Autodesk Fusion 360 part; units mm, degrees
(part 18 of 21)
  spline S78 degree 5 poles (9.9022, -20.7593) (9.9022, -20.752) (9.9024, -20.7374) (9.9025, -20.7155) (9.9026, -20.6864) (9.9026, -20.65) (9.9024, -20.6137) (9.9021, -20.5774) (9.9017, -20.5411) (9.9011, -20.5049) (9.9004, -20.4687) (9.8996, -20.4326) (9.8986, -20.3965) (9.8975, -20.3604) (9.8963, -20.3244) (9.8949, -20.2885) (9.8934, -20.2525) (9.8917, -20.2167) (9.8899, -20.1808) (9.8879, -20.145) (9.8858, -20.1093) (9.8836, -20.0736) (9.8812, -20.038) (9.8786, -20.0024) (9.8759, -19.9668) (9.8731, -19.9313) (9.8701, -19.8959) (9.867, -19.8605) (9.8637, -19.8252) (9.8602, -19.7899) (9.8566, -19.7547) (9.8529, -19.7195) (9.8489, -19.6844) (9.8449, -19.6493) (9.8406, -19.6143) (9.8362, -19.5794) (9.8316, -19.5445) (9.8269, -19.5097) (9.822, -19.4749) (9.8169, -19.4402) (9.8117, -19.4056) (9.8063, -19.3711) (9.8007, -19.3366) (9.7949, -19.3021) (9.789, -19.2678) (9.7828, -19.2335) (9.7765, -19.1993) (9.77, -19.1652) (9.7633, -19.1311) (9.7564, -19.0972) (9.7493, -19.0633) (9.742, -19.0295) (9.7345, -18.9957) (9.7268, -18.9621) (9.7189, -18.9286) (9.7108, -18.8951) (9.7024, -18.8618) (9.6938, -18.8285) (9.685, -18.7954) (9.6759, -18.7624) (9.6665, -18.7294) (9.6569, -18.6966) (9.6471, -18.6639) (9.637, -18.6313) (9.6266, -18.5989) (9.6158, -18.5666) (9.6066, -18.54) (9.5994, -18.5199) (9.5944, -18.5063) (9.5917, -18.499) (9.5913, -18.4981) knots -1 -1 -1 -1 -1 -1 -0.98571429 -0.97142857 -0.95714286 -0.94285714 -0.92857143 -0.91428571 -0.9 -0.88571429 -0.87142857 -0.85714286 -0.84285714 -0.82857143 -0.81428571 -0.8 -0.78571429 -0.77142857 -0.75714286 -0.74285714 -0.72857143 -0.71428571 -0.7 -0.68571429 -0.67142857 -0.65714286 -0.64285714 -0.62857143 -0.61428571 -0.6 -0.58571429 -0.57142857 -0.55714286 -0.54285714 -0.52857143 -0.51428571 -0.5 -0.48571429 -0.47142857 -0.45714286 -0.44285714 -0.42857143 -0.41428571 -0.4 -0.38571429 -0.37142857 -0.35714286 -0.34285714 -0.32857143 -0.31428571 -0.3 -0.28571429 -0.27142857 -0.25714286 -0.24285714 -0.22857143 -0.21428571 -0.2 -0.18571429 -0.17142857 -0.15714286 -0.14285714 -0.12857143 -0.11428571 -0.1 -0.08571429 -0.07142857 -0.06937658 -0.06937658 -0.06937658 -0.06937658 -0.06937658 -0.06937658
  spline S79 degree 3 poles (9.6386, -18.3746) (9.6271, -18.3807) (9.6168, -18.3889) (9.6001, -18.4089) (9.5937, -18.4204) (9.5864, -18.4434) (9.5848, -18.4545) (9.5853, -18.4767) (9.5875, -18.4877) (9.5913, -18.4981) knots 0 0 0 0 0.003906 0.003906 0.007813 0.007813 0.011148 0.011148 0.014483 0.014483 0.014483 0.014483
  arc A70 (9.6386, -18.3746) -> (10.2467, -18.0426) centre (0, 0) ccw
  spline S80 degree 3 poles (10.3761, -18.0696) (10.3683, -18.0592) (10.3585, -18.0504) (10.3362, -18.037) (10.3238, -18.0326) (10.2999, -18.029) (10.2887, -18.0292) (10.2669, -18.0332) (10.2564, -18.0371) (10.2467, -18.0426) knots 0 0 0 0 0.003906 0.003906 0.007813 0.007813 0.011148 0.011148 0.014483 0.014483 0.014483 0.014483
  spline S81 degree 5 poles (10.3761, -18.0696) (10.3767, -18.0704) (10.3813, -18.0766) (10.3901, -18.0882) (10.4031, -18.1051) (10.4205, -18.1272) (10.4419, -18.1537) (10.4635, -18.18) (10.4855, -18.2061) (10.5077, -18.2321) (10.5301, -18.2579) (10.5527, -18.2835) (10.5756, -18.3091) (10.5987, -18.3344) (10.622, -18.3596) (10.6455, -18.3847) (10.6693, -18.4096) (10.6932, -18.4344) (10.7173, -18.4591) (10.7417, -18.4836) (10.7662, -18.508) (10.7908, -18.5323) (10.8157, -18.5565) (10.8407, -18.5805) (10.8659, -18.6045) (10.8913, -18.6283) (10.9168, -18.652) (10.9425, -18.6755) (10.9683, -18.699) (10.9943, -18.7223) (11.0204, -18.7456) (11.0467, -18.7687) (11.0732, -18.7917) (11.0998, -18.8147) (11.1265, -18.8375) (11.1534, -18.8602) (11.1804, -18.8828) (11.2075, -18.9052) (11.2348, -18.9276) (11.2622, -18.9499) (11.2898, -18.9721) (11.3175, -18.9942) (11.3453, -19.0161) (11.3732, -19.038) (11.4013, -19.0598) (11.4295, -19.0815) (11.4578, -19.1031) (11.4863, -19.1245) (11.5149, -19.1459) (11.5435, -19.1672) (11.5724, -19.1884) (11.6013, -19.2095) (11.6303, -19.2305) (11.6595, -19.2514) (11.6888, -19.2722) (11.7182, -19.2929) (11.7477, -19.3135) (11.7773, -19.334) (11.807, -19.3544) (11.8369, -19.3748) (11.8668, -19.395) (11.8969, -19.4152) (11.927, -19.4352) (11.9573, -19.4552) (11.9877, -19.475) (12.0182, -19.4948) (12.0488, -19.5145) (12.0733, -19.5302) (12.0918, -19.5419) (12.1041, -19.5497) (12.1103, -19.5535) knots 0.06937658 0.06937658 0.06937658 0.06937658 0.06937658 0.06937658 0.07142857 0.08571429 0.1 0.11428571 0.12857143 0.14285714 0.15714286 0.17142857 0.18571429 0.2 0.21428571 0.22857143 0.24285714 0.25714286 0.27142857 0.28571429 0.3 0.31428571 0.32857143 0.34285714 0.35714286 0.37142857 0.38571429 0.4 0.41428571 0.42857143 0.44285714 0.45714286 0.47142857 0.48571429 0.5 0.51428571 0.52857143 0.54285714 0.55714286 0.57142857 0.58571429 0.6 0.61428571 0.62857143 0.64285714 0.65714286 0.67142857 0.68571429 0.7 0.71428571 0.72857143 0.74285714 0.75714286 0.77142857 0.78571429 0.8 0.81428571 0.82857143 0.84285714 0.85714286 0.87142857 0.88571429 0.9 0.91428571 0.92857143 0.94285714 0.95714286 0.97142857 0.98571429 1 1 1 1 1 1
  arc A71 (12.1103, -19.5535) -> (12.7557, -19.1387) centre (0, 0) ccw
  spline S82 degree 5 poles (12.7557, -19.1387) (12.7548, -19.1315) (12.7528, -19.1171) (12.7498, -19.0954) (12.7458, -19.0665) (12.7406, -19.0305) (12.7352, -18.9946) (12.7298, -18.9587) (12.7242, -18.9229) (12.7185, -18.8871) (12.7127, -18.8514) (12.7067, -18.8158) (12.7006, -18.7802) (12.6944, -18.7446) (12.688, -18.7092) (12.6815, -18.6738) (12.6749, -18.6384) (12.6681, -18.6032) (12.6612, -18.5679) (12.6542, -18.5328) (12.647, -18.4977) (12.6397, -18.4627) (12.6323, -18.4278) (12.6247, -18.3929) (12.617, -18.3581) (12.6091, -18.3234) (12.6011, -18.2887) (12.593, -18.2541) (12.5847, -18.2196) (12.5763, -18.1852) (12.5677, -18.1509) (12.5589, -18.1166) (12.5501, -18.0824) (12.541, -18.0483) (12.5319, -18.0142) (12.5225, -17.9803) (12.513, -17.9464) (12.5034, -17.9126) (12.4936, -17.8789) (12.4836, -17.8453) (12.4735, -17.8117) (12.4633, -17.7783) (12.4528, -17.745) (12.4422, -17.7117) (12.4314, -17.6786) (12.4205, -17.6455) (12.4094, -17.6125) (12.3981, -17.5797) (12.3866, -17.5469) (12.3749, -17.5143) (12.3631, -17.4818) (12.351, -17.4493) (12.3388, -17.417) (12.3264, -17.3848) (12.3138, -17.3527) (12.301, -17.3208) (12.288, -17.289) (12.2747, -17.2573) (12.2612, -17.2258) (12.2475, -17.1944) (12.2336, -17.1631) (12.2194, -17.132) (12.205, -17.101) (12.1904, -17.0702) (12.1755, -17.0396) (12.1602, -17.0092) (12.1473, -16.9841) (12.1374, -16.9653) (12.1304, -16.9525) (12.1267, -16.9457) (12.1263, -16.9448) knots -1 -1 -1 -1 -1 -1 -0.98571429 -0.97142857 -0.95714286 -0.94285714 -0.92857143 -0.91428571 -0.9 -0.88571429 -0.87142857 -0.85714286 -0.84285714 -0.82857143 -0.81428571 -0.8 -0.78571429 -0.77142857 -0.75714286 -0.74285714 -0.72857143 -0.71428571 -0.7 -0.68571429 -0.67142857 -0.65714286 -0.64285714 -0.62857143 -0.61428571 -0.6 -0.58571429 -0.57142857 -0.55714286 -0.54285714 -0.52857143 -0.51428571 -0.5 -0.48571429 -0.47142857 -0.45714286 -0.44285714 -0.42857143 -0.41428571 -0.4 -0.38571429 -0.37142857 -0.35714286 -0.34285714 -0.32857143 -0.31428571 -0.3 -0.28571429 -0.27142857 -0.25714286 -0.24285714 -0.22857143 -0.21428571 -0.2 -0.18571429 -0.17142857 -0.15714286 -0.14285714 -0.12857143 -0.11428571 -0.1 -0.08571429 -0.07142857 -0.06937658 -0.06937658 -0.06937658 -0.06937658 -0.06937658 -0.06937658
  spline S83 degree 3 poles (12.1555, -16.8159) (12.1449, -16.8235) (12.136, -16.8331) (12.1222, -16.8552) (12.1176, -16.8675) (12.1136, -16.8914) (12.1136, -16.9025) (12.1173, -16.9245) (12.1209, -16.9351) (12.1263, -16.9448) knots 0 0 0 0 0.003906 0.003906 0.007813 0.007813 0.011148 0.011148 0.014483 0.014483 0.014483 0.014483
  arc A72 (12.1555, -16.8159) -> (12.7101, -16.4007) centre (0, 0) ccw
  spline S84 degree 3 poles (12.8421, -16.409) (12.8329, -16.3998) (12.8219, -16.3925) (12.7979, -16.3824) (12.785, -16.3798) (12.7609, -16.3796) (12.7498, -16.3814) (12.7288, -16.3886) (12.7189, -16.3939) (12.7101, -16.4007) knots 0 0 0 0 0.003906 0.003906 0.007813 0.007813 0.011148 0.011148 0.014483 0.014483 0.014483 0.014483
  spline S85 degree 5 poles (12.8421, -16.409) (12.8428, -16.4097) (12.8482, -16.4151) (12.8586, -16.4254) (12.8739, -16.4403) (12.8942, -16.4597) (12.9191, -16.4829) (12.9443, -16.5058) (12.9698, -16.5286) (12.9954, -16.5511) (13.0213, -16.5735) (13.0473, -16.5956) (13.0736, -16.6176) (13.1001, -16.6394) (13.1267, -16.6611) (13.1536, -16.6826) (13.1806, -16.7039) (13.2079, -16.725) (13.2353, -16.746) (13.2628, -16.7668) (13.2905, -16.7875) (13.3184, -16.808) (13.3465, -16.8284) (13.3747, -16.8486) (13.403, -16.8687) (13.4315, -16.8887) (13.4601, -16.9085) (13.4889, -16.9282) (13.5178, -16.9477) (13.5469, -16.9671) (13.576, -16.9864) (13.6054, -17.0056) (13.6348, -17.0246) (13.6644, -17.0435) (13.6941, -17.0623) (13.7239, -17.0809) (13.7539, -17.0994) (13.784, -17.1178) (13.8141, -17.1361) (13.8445, -17.1542) (13.8749, -17.1723) (13.9054, -17.1902) (13.9361, -17.208) (13.9669, -17.2257) (13.9978, -17.2432) (14.0288, -17.2607) (14.0599, -17.278) (14.0911, -17.2952) (14.1224, -17.3123) (14.1538, -17.3293) (14.1854, -17.3462) (14.217, -17.3629) (14.2487, -17.3796) (14.2806, -17.3961) (14.3125, -17.4125) (14.3446, -17.4288) (14.3767, -17.445) (14.4089, -17.4611) (14.4413, -17.4771) (14.4737, -17.493) (14.5062, -17.5088) (14.5388, -17.5244) (14.5715, -17.54) (14.6044, -17.5554) (14.6373, -17.5708) (14.6702, -17.586) (14.7033, -17.6011) (14.7299, -17.6132) (14.7498, -17.6221) (14.7631, -17.6281) (14.7698, -17.631) knots 0.06937658 0.06937658 0.06937658 0.06937658 0.06937658 0.06937658 0.07142857 0.08571429 0.1 0.11428571 0.12857143 0.14285714 0.15714286 0.17142857 0.18571429 0.2 0.21428571 0.22857143 0.24285714 0.25714286 0.27142857 0.28571429 0.3 0.31428571 0.32857143 0.34285714 0.35714286 0.37142857 0.38571429 0.4 0.41428571 0.42857143 0.44285714 0.45714286 0.47142857 0.48571429 0.5 0.51428571 0.52857143 0.54285714 0.55714286 0.57142857 0.58571429 0.6 0.61428571 0.62857143 0.64285714 0.65714286 0.67142857 0.68571429 0.7 0.71428571 0.72857143 0.74285714 0.75714286 0.77142857 0.78571429 0.8 0.81428571 0.82857143 0.84285714 0.85714286 0.87142857 0.88571429 0.9 0.91428571 0.92857143 0.94285714 0.95714286 0.97142857 0.98571429 1 1 1 1 1 1
  arc A73 (14.7698, -17.631) -> (15.3496, -17.1286) centre (0, 0) ccw
  spline S86 degree 5 poles (15.3496, -17.1286) (15.3476, -17.1216) (15.3436, -17.1076) (15.3376, -17.0865) (15.3295, -17.0586) (15.3192, -17.0237) (15.3088, -16.9888) (15.2983, -16.9541) (15.2877, -16.9194) (15.277, -16.8848) (15.2661, -16.8503) (15.2551, -16.8159) (15.244, -16.7815) (15.2328, -16.7472) (15.2215, -16.713) (15.21, -16.6789) (15.1984, -16.6449) (15.1867, -16.6109) (15.1749, -16.5771) (15.1629, -16.5433) (15.1508, -16.5096) (15.1386, -16.476) (15.1263, -16.4425) (15.1138, -16.409) (15.1012, -16.3757) (15.0885, -16.3424) (15.0756, -16.3093) (15.0626, -16.2762) (15.0495, -16.2432) (15.0363, -16.2103) (15.0229, -16.1775) (15.0094, -16.1448) (14.9957, -16.1123) (14.9819, -16.0798) (14.968, -16.0474) (14.9539, -16.0151) (14.9397, -15.9829) (14.9254, -15.9508) (14.9109, -15.9189) (14.8962, -15.887) (14.8814, -15.8553) (14.8665, -15.8236) (14.8514, -15.7921) (14.8362, -15.7607) (14.8208, -15.7294) (14.8053, -15.6983) (14.7896, -15.6672) (14.7737, -15.6363) (14.7577, -15.6055) (14.7415, -15.5749) (14.7252, -15.5444) (14.7086, -15.514) (14.6919, -15.4837) (14.6751, -15.4536) (14.658, -15.4237) (14.6408, -15.3939) (14.6234, -15.3642) (14.6057, -15.3348) (14.5879, -15.3055) (14.5699, -15.2763) (14.5516, -15.2474) (14.5332, -15.2186) (14.5145, -15.19) (14.4957, -15.1616) (14.4765, -15.1334) (14.4571, -15.1054) (14.4408, -15.0825) (14.4282, -15.0653) (14.4196, -15.0536) (14.4149, -15.0474) (14.4143, -15.0466) knots -1 -1 -1 -1 -1 -1 -0.98571429 -0.97142857 -0.95714286 -0.94285714 -0.92857143 -0.91428571 -0.9 -0.88571429 -0.87142857 -0.85714286 -0.84285714 -0.82857143 -0.81428571 -0.8 -0.78571429 -0.77142857 -0.75714286 -0.74285714 -0.72857143 -0.71428571 -0.7 -0.68571429 -0.67142857 -0.65714286 -0.64285714 -0.62857143 -0.61428571 -0.6 -0.58571429 -0.57142857 -0.55714286 -0.54285714 -0.52857143 -0.51428571 -0.5 -0.48571429 -0.47142857 -0.45714286 -0.44285714 -0.42857143 -0.41428571 -0.4 -0.38571429 -0.37142857 -0.35714286 -0.34285714 -0.32857143 -0.31428571 -0.3 -0.28571429 -0.27142857 -0.25714286 -0.24285714 -0.22857143 -0.21428571 -0.2 -0.18571429 -0.17142857 -0.15714286 -0.14285714 -0.12857143 -0.11428571 -0.1 -0.08571429 -0.07142857 -0.06937658 -0.06937658 -0.06937658 -0.06937658 -0.06937658 -0.06937658
  spline S87 degree 3 poles (14.4249, -14.9148) (14.4155, -14.9239) (14.408, -14.9347) (14.3976, -14.9585) (14.3947, -14.9713) (14.3942, -14.9955) (14.3958, -15.0066) (14.4026, -15.0277) (14.4077, -15.0377) (14.4143, -15.0466) knots 0 0 0 0 0.003906 0.003906 0.007813 0.007813 0.011148 0.011148 0.014483 0.014483 0.014483 0.014483
  arc A74 (14.4249, -14.9148) -> (14.9148, -14.4249) centre (0, 0) ccw
  spline S88 degree 3 poles (15.0466, -14.4143) (15.0362, -14.4065) (15.0243, -14.4009) (14.9991, -14.3943) (14.986, -14.3936) (14.9621, -14.3969) (14.9514, -14.4002) (14.9315, -14.4103) (14.9225, -14.4169) (14.9148, -14.4249) knots 0 0 0 0 0.003906 0.003906 0.007813 0.007813 0.011148 0.011148 0.014483 0.014483 0.014483 0.014483
  spline S89 degree 5 poles (15.0466, -14.4143) (15.0474, -14.4149) (15.0536, -14.4196) (15.0653, -14.4282) (15.0825, -14.4408) (15.1054, -14.4571) (15.1334, -14.4765) (15.1616, -14.4957) (15.19, -14.5145) (15.2186, -14.5332) (15.2474, -14.5516) (15.2763, -14.5699) (15.3055, -14.5879) (15.3348, -14.6057) (15.3642, -14.6234) (15.3939, -14.6408) (15.4237, -14.658) (15.4536, -14.6751) (15.4837, -14.6919) (15.514, -14.7086) (15.5444, -14.7252) (15.5749, -14.7415) (15.6055, -14.7577) (15.6363, -14.7737) (15.6672, -14.7896) (15.6983, -14.8053) (15.7294, -14.8208) (15.7607, -14.8362) (15.7921, -14.8514) (15.8236, -14.8665) (15.8553, -14.8814) (15.887, -14.8962) (15.9189, -14.9109) (15.9508, -14.9254) (15.9829, -14.9397) (16.0151, -14.9539) (16.0474, -14.968) (16.0798, -14.9819) (16.1123, -14.9957) (16.1448, -15.0094) (16.1775, -15.0229) (16.2103, -15.0363) (16.2432, -15.0495) (16.2762, -15.0626) (16.3093, -15.0756) (16.3424, -15.0885) (16.3757, -15.1012) (16.409, -15.1138) (16.4425, -15.1263) (16.476, -15.1386) (16.5096, -15.1508) (16.5433, -15.1629) (16.5771, -15.1749) (16.6109, -15.1867) (16.6449, -15.1984) (16.6789, -15.21) (16.713, -15.2215) (16.7472, -15.2328) (16.7815, -15.244) (16.8159, -15.2551) (16.8503, -15.2661) (16.8848, -15.277) (16.9194, -15.2877) (16.9541, -15.2983) (16.9888, -15.3088) (17.0237, -15.3192) (17.0586, -15.3295) (17.0865, -15.3376) (17.1076, -15.3436) (17.1216, -15.3476) (17.1286, -15.3496) knots 0.06937658 0.06937658 0.06937658 0.06937658 0.06937658 0.06937658 0.07142857 0.08571429 0.1 0.11428571 0.12857143 0.14285714 0.15714286 0.17142857 0.18571429 0.2 0.21428571 0.22857143 0.24285714 0.25714286 0.27142857 0.28571429 0.3 0.31428571 0.32857143 0.34285714 0.35714286 0.37142857 0.38571429 0.4 0.41428571 0.42857143 0.44285714 0.45714286 0.47142857 0.48571429 0.5 0.51428571 0.52857143 0.54285714 0.55714286 0.57142857 0.58571429 0.6 0.61428571 0.62857143 0.64285714 0.65714286 0.67142857 0.68571429 0.7 0.71428571 0.72857143 0.74285714 0.75714286 0.77142857 0.78571429 0.8 0.81428571 0.82857143 0.84285714 0.85714286 0.87142857 0.88571429 0.9 0.91428571 0.92857143 0.94285714 0.95714286 0.97142857 0.98571429 1 1 1 1 1 1
  arc A75 (17.1286, -15.3496) -> (17.631, -14.7698) centre (0, 0) ccw
  spline S90 degree 5 poles (17.631, -14.7698) (17.6281, -14.7631) (17.6221, -14.7498) (17.6132, -14.7299) (17.6011, -14.7033) (17.586, -14.6702) (17.5708, -14.6373) (17.5554, -14.6044) (17.54, -14.5715) (17.5244, -14.5388) (17.5088, -14.5062) (17.493, -14.4737) (17.4771, -14.4413) (17.4611, -14.4089) (17.445, -14.3767) (17.4288, -14.3446) (17.4125, -14.3125) (17.3961, -14.2806) (17.3796, -14.2487) (17.3629, -14.217) (17.3462, -14.1854) (17.3293, -14.1538) (17.3123, -14.1224) (17.2952, -14.0911) (17.278, -14.0599) (17.2607, -14.0288) (17.2432, -13.9978) (17.2257, -13.9669) (17.208, -13.9361) (17.1902, -13.9054) (17.1723, -13.8749) (17.1542, -13.8445) (17.1361, -13.8141) (17.1178, -13.784) (17.0994, -13.7539) (17.0809, -13.7239) (17.0623, -13.6941) (17.0435, -13.6644) (17.0246, -13.6348) (17.0056, -13.6054) (16.9864, -13.576) (16.9671, -13.5469) (16.9477, -13.5178) (16.9282, -13.4889) (16.9085, -13.4601) (16.8887, -13.4315) (16.8687, -13.403) (16.8486, -13.3747) (16.8284, -13.3465) (16.808, -13.3184) (16.7875, -13.2905) (16.7668, -13.2628) (16.746, -13.2353) (16.725, -13.2079) (16.7039, -13.1806) (16.6826, -13.1536) (16.6611, -13.1267) (16.6394, -13.1001) (16.6176, -13.0736) (16.5956, -13.0473) (16.5735, -13.0213) (16.5511, -12.9954) (16.5286, -12.9698) (16.5058, -12.9443) (16.4829, -12.9191) (16.4597, -12.8942) (16.4403, -12.8739) (16.4254, -12.8586) (16.4151, -12.8482) (16.4097, -12.8428) (16.409, -12.8421) knots -1 -1 -1 -1 -1 -1 -0.98571429 -0.97142857 -0.95714286 -0.94285714 -0.92857143 -0.91428571 -0.9 -0.88571429 -0.87142857 -0.85714286 -0.84285714 -0.82857143 -0.81428571 -0.8 -0.78571429 -0.77142857 -0.75714286 -0.74285714 -0.72857143 -0.71428571 -0.7 -0.68571429 -0.67142857 -0.65714286 -0.64285714 -0.62857143 -0.61428571 -0.6 -0.58571429 -0.57142857 -0.55714286 -0.54285714 -0.52857143 -0.51428571 -0.5 -0.48571429 -0.47142857 -0.45714286 -0.44285714 -0.42857143 -0.41428571 -0.4 -0.38571429 -0.37142857 -0.35714286 -0.34285714 -0.32857143 -0.31428571 -0.3 -0.28571429 -0.27142857 -0.25714286 -0.24285714 -0.22857143 -0.21428571 -0.2 -0.18571429 -0.17142857 -0.15714286 -0.14285714 -0.12857143 -0.11428571 -0.1 -0.08571429 -0.07142857 -0.06937658 -0.06937658 -0.06937658 -0.06937658 -0.06937658 -0.06937658
  spline S91 degree 3 poles (16.4007, -12.7101) (16.3927, -12.7204) (16.3868, -12.7322) (16.3799, -12.7573) (16.3789, -12.7704) (16.3818, -12.7943) (16.3849, -12.8051) (16.3946, -12.8251) (16.4011, -12.8342) (16.409, -12.8421) knots 0 0 0 0 0.003906 0.003906 0.007813 0.007813 0.011148 0.011148 0.014483 0.014483 0.014483 0.014483
  arc A76 (16.4007, -12.7101) -> (16.8159, -12.1555) centre (0, 0) ccw
  spline S92 degree 3 poles (16.9448, -12.1263) (16.9334, -12.12) (16.9208, -12.1161) (16.895, -12.1132) (16.8819, -12.1143) (16.8587, -12.121) (16.8486, -12.1258) (16.8304, -12.1386) (16.8224, -12.1465) (16.8159, -12.1555) knots 0 0 0 0 0.003906 0.003906 0.007813 0.007813 0.011148 0.011148 0.014483 0.014483 0.014483 0.014483
  spline S93 degree 5 poles (16.9448, -12.1263) (16.9457, -12.1267) (16.9525, -12.1304) (16.9653, -12.1374) (16.9841, -12.1473) (17.0092, -12.1602) (17.0396, -12.1755) (17.0702, -12.1904) (17.101, -12.205) (17.132, -12.2194) (17.1631, -12.2336) (17.1944, -12.2475) (17.2258, -12.2612) (17.2573, -12.2747) (17.289, -12.288) (17.3208, -12.301) (17.3527, -12.3138) (17.3848, -12.3264) (17.417, -12.3388) (17.4493, -12.351) (17.4818, -12.3631) (17.5143, -12.3749) (17.5469, -12.3866) (17.5797, -12.3981) (17.6125, -12.4094) (17.6455, -12.4205) (17.6786, -12.4314) (17.7117, -12.4422) (17.745, -12.4528) (17.7783, -12.4633) (17.8117, -12.4735) (17.8453, -12.4836) (17.8789, -12.4936) (17.9126, -12.5034) (17.9464, -12.513) (17.9803, -12.5225) (18.0142, -12.5319) (18.0483, -12.541) (18.0824, -12.5501) (18.1166, -12.5589) (18.1509, -12.5677) (18.1852, -12.5763) (18.2196, -12.5847) (18.2541, -12.593) (18.2887, -12.6011) (18.3234, -12.6091) (18.3581, -12.617) (18.3929, -12.6247) (18.4278, -12.6323) (18.4627, -12.6397) (18.4977, -12.647) (18.5328, -12.6542) (18.5679, -12.6612) (18.6032, -12.6681) (18.6384, -12.6749) (18.6738, -12.6815) (18.7092, -12.688) (18.7446, -12.6944) (18.7802, -12.7006) (18.8158, -12.7067) (18.8514, -12.7127) (18.8871, -12.7185) (18.9229, -12.7242) (18.9587, -12.7298) (18.9946, -12.7352) (19.0305, -12.7406) (19.0665, -12.7458) (19.0954, -12.7498) (19.1171, -12.7528) (19.1315, -12.7548) (19.1387, -12.7557) knots 0.06937658 0.06937658 0.06937658 0.06937658 0.06937658 0.06937658 0.07142857 0.08571429 0.1 0.11428571 0.12857143 0.14285714 0.15714286 0.17142857 0.18571429 0.2 0.21428571 0.22857143 0.24285714 0.25714286 0.27142857 0.28571429 0.3 0.31428571 0.32857143 0.34285714 0.35714286 0.37142857 0.38571429 0.4 0.41428571 0.42857143 0.44285714 0.45714286 0.47142857 0.48571429 0.5 0.51428571 0.52857143 0.54285714 0.55714286 0.57142857 0.58571429 0.6 0.61428571 0.62857143 0.64285714 0.65714286 0.67142857 0.68571429 0.7 0.71428571 0.72857143 0.74285714 0.75714286 0.77142857 0.78571429 0.8 0.81428571 0.82857143 0.84285714 0.85714286 0.87142857 0.88571429 0.9 0.91428571 0.92857143 0.94285714 0.95714286 0.97142857 0.98571429 1 1 1 1 1 1
  arc A77 (19.1387, -12.7557) -> (19.5535, -12.1103) centre (0, 0) ccw
  spline S94 degree 5 poles (19.5535, -12.1103) (19.5497, -12.1041) (19.5419, -12.0918) (19.5302, -12.0733) (19.5145, -12.0488) (19.4948, -12.0182) (19.475, -11.9877) (19.4552, -11.9573) (19.4352, -11.927) (19.4152, -11.8969) (19.395, -11.8668) (19.3748, -11.8369) (19.3544, -11.807) (19.334, -11.7773) (19.3135, -11.7477) (19.2929, -11.7182) (19.2722, -11.6888) (19.2514, -11.6595) (19.2305, -11.6303) (19.2095, -11.6013) (19.1884, -11.5724) (19.1672, -11.5435) (19.1459, -11.5149) (19.1245, -11.4863) (19.1031, -11.4578) (19.0815, -11.4295) (19.0598, -11.4013) (19.038, -11.3732) (19.0161, -11.3453) (18.9942, -11.3175) (18.9721, -11.2898) (18.9499, -11.2622) (18.9276, -11.2348) (18.9052, -11.2075) (18.8828, -11.1804) (18.8602, -11.1534) (18.8375, -11.1265) (18.8147, -11.0998) (18.7917, -11.0732) (18.7687, -11.0467) (18.7456, -11.0204) (18.7223, -10.9943) (18.699, -10.9683) (18.6755, -10.9425) (18.652, -10.9168) (18.6283, -10.8913) (18.6045, -10.8659) (18.5805, -10.8407) (18.5565, -10.8157) (18.5323, -10.7908) (18.508, -10.7662) (18.4836, -10.7417) (18.4591, -10.7173) (18.4344, -10.6932) (18.4096, -10.6693) (18.3847, -10.6455) (18.3596, -10.622) (18.3344, -10.5987) (18.3091, -10.5756) (18.2835, -10.5527) (18.2579, -10.5301) (18.2321, -10.5077) (18.2061, -10.4855) (18.18, -10.4635) (18.1537, -10.4419) (18.1272, -10.4205) (18.1051, -10.4031) (18.0882, -10.3901) (18.0766, -10.3813) (18.0704, -10.3767) (18.0696, -10.3761) knots -1 -1 -1 -1 -1 -1 -0.98571429 -0.97142857 -0.95714286 -0.94285714 -0.92857143 -0.91428571 -0.9 -0.88571429 -0.87142857 -0.85714286 -0.84285714 -0.82857143 -0.81428571 -0.8 -0.78571429 -0.77142857 -0.75714286 -0.74285714 -0.72857143 -0.71428571 -0.7 -0.68571429 -0.67142857 -0.65714286 -0.64285714 -0.62857143 -0.61428571 -0.6 -0.58571429 -0.57142857 -0.55714286 -0.54285714 -0.52857143 -0.51428571 -0.5 -0.48571429 -0.47142857 -0.45714286 -0.44285714 -0.42857143 -0.41428571 -0.4 -0.38571429 -0.37142857 -0.35714286 -0.34285714 -0.32857143 -0.31428571 -0.3 -0.28571429 -0.27142857 -0.25714286 -0.24285714 -0.22857143 -0.21428571 -0.2 -0.18571429 -0.17142857 -0.15714286 -0.14285714 -0.12857143 -0.11428571 -0.1 -0.08571429 -0.07142857 -0.06937658 -0.06937658 -0.06937658 -0.06937658 -0.06937658 -0.06937658
  spline S95 degree 3 poles (18.0426, -10.2467) (18.0361, -10.258) (18.032, -10.2705) (18.0287, -10.2963) (18.0296, -10.3094) (18.0358, -10.3327) (18.0405, -10.3429) (18.053, -10.3613) (18.0607, -10.3694) (18.0696, -10.3761) knots 0 0 0 0 0.003906 0.003906 0.007813 0.007813 0.011148 0.011148 0.014483 0.014483 0.014483 0.014483
  arc A78 (18.0426, -10.2467) -> (18.3746, -9.6386) centre (0, 0) ccw
  spline S96 degree 3 poles (18.4981, -9.5913) (18.4859, -9.5868) (18.4729, -9.5847) (18.4469, -9.5855) (18.4341, -9.5885) (18.4121, -9.5984) (18.4027, -9.6046) (18.3866, -9.6198) (18.3798, -9.6288) (18.3746, -9.6386) knots 0 0 0 0 0.003906 0.003906 0.007813 0.007813 0.011148 0.011148 0.014483 0.014483 0.014483 0.014483
  spline S97 degree 5 poles (18.4981, -9.5913) (18.499, -9.5917) (18.5063, -9.5944) (18.5199, -9.5994) (18.54, -9.6066) (18.5666, -9.6158) (18.5989, -9.6266) (18.6313, -9.637) (18.6639, -9.6471) (18.6966, -9.6569) (18.7294, -9.6665) (18.7624, -9.6759) (18.7954, -9.685) (18.8285, -9.6938) (18.8618, -9.7024) (18.8951, -9.7108) (18.9286, -9.7189) (18.9621, -9.7268) (18.9957, -9.7345) (19.0295, -9.742) (19.0633, -9.7493) (19.0972, -9.7564) (19.1311, -9.7633) (19.1652, -9.77) (19.1993, -9.7765) (19.2335, -9.7828) (19.2678, -9.789) (19.3021, -9.7949) (19.3366, -9.8007) (19.3711, -9.8063) (19.4056, -9.8117) (19.4402, -9.8169) (19.4749, -9.822) (19.5097, -9.8269) (19.5445, -9.8316) (19.5794, -9.8362) (19.6143, -9.8406) (19.6493, -9.8449) (19.6844, -9.8489) (19.7195, -9.8529) (19.7547, -9.8566) (19.7899, -9.8602) (19.8252, -9.8637) (19.8605, -9.867) (19.8959, -9.8701) (19.9313, -9.8731) (19.9668, -9.8759) (20.0024, -9.8786) (20.038, -9.8812) (20.0736, -9.8836) (20.1093, -9.8858) (20.145, -9.8879) (20.1808, -9.8899) (20.2167, -9.8917) (20.2525, -9.8934) (20.2885, -9.8949) (20.3244, -9.8963) (20.3604, -9.8975) (20.3965, -9.8986) (20.4326, -9.8996) (20.4687, -9.9004) (20.5049, -9.9011) (20.5411, -9.9017) (20.5774, -9.9021) (20.6137, -9.9024) (20.65, -9.9026) (20.6864, -9.9026) (20.7155, -9.9025) (20.7374, -9.9024) (20.752, -9.9022) (20.7593, -9.9022) knots 0.06937658 0.06937658 0.06937658 0.06937658 0.06937658 0.06937658 0.07142857 0.08571429 0.1 0.11428571 0.12857143 0.14285714 0.15714286 0.17142857 0.18571429 0.2 0.21428571 0.22857143 0.24285714 0.25714286 0.27142857 0.28571429 0.3 0.31428571 0.32857143 0.34285714 0.35714286 0.37142857 0.38571429 0.4 0.41428571 0.42857143 0.44285714 0.45714286 0.47142857 0.48571429 0.5 0.51428571 0.52857143 0.54285714 0.55714286 0.57142857 0.58571429 0.6 0.61428571 0.62857143 0.64285714 0.65714286 0.67142857 0.68571429 0.7 0.71428571 0.72857143 0.74285714 0.75714286 0.77142857 0.78571429 0.8 0.81428571 0.82857143 0.84285714 0.85714286 0.87142857 0.88571429 0.9 0.91428571 0.92857143 0.94285714 0.95714286 0.97142857 0.98571429 1 1 1 1 1 1
  arc A79 (20.7593, -9.9022) -> (21.078, -9.2043) centre (0, 0) ccw
  spline S98 degree 5 poles (21.078, -9.2043) (21.0733, -9.1987) (21.0638, -9.1876) (21.0496, -9.171) (21.0306, -9.1489) (21.0067, -9.1214) (20.9828, -9.0941) (20.9588, -9.0668) (20.9348, -9.0397) (20.9106, -9.0127) (20.8864, -8.9858) (20.8621, -8.9591) (20.8378, -8.9324) (20.8133, -8.9059) (20.7888, -8.8795) (20.7642, -8.8532) (20.7395, -8.8271) (20.7147, -8.8011) (20.6899, -8.7752) (20.665, -8.7494) (20.64, -8.7238) (20.6149, -8.6983) (20.5898, -8.6729) (20.5645, -8.6477) (20.5392, -8.6226) (20.5138, -8.5976) (20.4884, -8.5728) (20.4628, -8.5481) (20.4372, -8.5235) (20.4115, -8.4991) (20.3857, -8.4749) (20.3598, -8.4508) (20.3339, -8.4268) (20.3078, -8.403) (20.2817, -8.3793) (20.2555, -8.3558) (20.2292, -8.3324) (20.2028, -8.3092) (20.1763, -8.2861) (20.1498, -8.2632) (20.1232, -8.2405) (20.0964, -8.2179) (20.0696, -8.1955) (20.0427, -8.1733) (20.0157, -8.1512) (19.9886, -8.1293) (19.9615, -8.1076) (19.9342, -8.0861) (19.9068, -8.0647) (19.8794, -8.0436) (19.8518, -8.0226) (19.8242, -8.0018) (19.7964, -7.9813) (19.7686, -7.9609) (19.7406, -7.9407) (19.7126, -7.9208) (19.6844, -7.901) (19.6561, -7.8816) (19.6278, -7.8623) (19.5993, -7.8433) (19.5706, -7.8245) (19.5419, -7.806) (19.513, -7.7878) (19.4841, -7.7698) (19.455, -7.7521) (19.4257, -7.7347) (19.4013, -7.7206) (19.3827, -7.7101) (19.37, -7.7031) (19.3632, -7.6994) (19.3623, -7.6989) knots -1 -1 -1 -1 -1 -1 -0.98571429 -0.97142857 -0.95714286 -0.94285714 -0.92857143 -0.91428571 -0.9 -0.88571429 -0.87142857 -0.85714286 -0.84285714 -0.82857143 -0.81428571 -0.8 -0.78571429 -0.77142857 -0.75714286 -0.74285714 -0.72857143 -0.71428571 -0.7 -0.68571429 -0.67142857 -0.65714286 -0.64285714 -0.62857143 -0.61428571 -0.6 -0.58571429 -0.57142857 -0.55714286 -0.54285714 -0.52857143 -0.51428571 -0.5 -0.48571429 -0.47142857 -0.45714286 -0.44285714 -0.42857143 -0.41428571 -0.4 -0.38571429 -0.37142857 -0.35714286 -0.34285714 -0.32857143 -0.31428571 -0.3 -0.28571429 -0.27142857 -0.25714286 -0.24285714 -0.22857143 -0.21428571 -0.2 -0.18571429 -0.17142857 -0.15714286 -0.14285714 -0.12857143 -0.11428571 -0.1 -0.08571429 -0.07142857 -0.06937658 -0.06937658 -0.06937658 -0.06937658 -0.06937658 -0.06937658
  spline S99 degree 3 poles (19.3172, -7.5747) (19.3124, -7.5868) (19.3101, -7.5997) (19.3105, -7.6258) (19.3132, -7.6386) (19.3228, -7.6608) (19.3288, -7.6702) (19.3438, -7.6867) (19.3526, -7.6936) (19.3623, -7.6989) knots 0 0 0 0 0.003906 0.003906 0.007813 0.007813 0.011148 0.011148 0.014483 0.014483 0.014483 0.014483
  arc A80 (19.3172, -7.5747) -> (19.5593, -6.9255) centre (0, 0) ccw
  spline S100 degree 3 poles (19.6748, -6.8612) (19.6621, -6.8584) (19.6489, -6.8582) (19.6233, -6.8627) (19.611, -6.8675) (19.5906, -6.8804) (19.5823, -6.8879) (19.5685, -6.9052) (19.563, -6.915) (19.5593, -6.9255) knots 0 0 0 0 0.003906 0.003906 0.007813 0.007813 0.011148 0.011148 0.014483 0.014483 0.014483 0.014483
  spline S101 degree 5 poles (19.6748, -6.8612) (19.6757, -6.8614) (19.6833, -6.863) (19.6975, -6.866) (19.7185, -6.8703) (19.7461, -6.8756) (19.7796, -6.8817) (19.8132, -6.8874) (19.8469, -6.8927) (19.8806, -6.8978) (19.9145, -6.9026) (19.9484, -6.9072) (19.9824, -6.9115) (20.0164, -6.9156) (20.0506, -6.9194) (20.0848, -6.9229) (20.119, -6.9262) (20.1534, -6.9292) (20.1878, -6.9321) (20.2222, -6.9347) (20.2567, -6.9371) (20.2913, -6.9393) (20.3259, -6.9413) (20.3605, -6.9431) (20.3952, -6.9447) (20.43, -6.9461) (20.4648, -6.9472) (20.4996, -6.9482) (20.5345, -6.9491) (20.5695, -6.9497) (20.6044, -6.9501) (20.6395, -6.9504) (20.6745, -6.9505) (20.7096, -6.9504) (20.7448, -6.9501) (20.7799, -6.9497) (20.8151, -6.949) (20.8504, -6.9483) (20.8857, -6.9473) (20.921, -6.9462) (20.9563, -6.9449) (20.9917, -6.9435) (21.0271, -6.9419) (21.0626, -6.9401) (21.0981, -6.9382) (21.1336, -6.9361) (21.1691, -6.9338) (21.2047, -6.9314) (21.2403, -6.9289) (21.2759, -6.9262) (21.3115, -6.9233) (21.3472, -6.9203) (21.3829, -6.9172) (21.4186, -6.9139) (21.4544, -6.9104) (21.4901, -6.9068) (21.5259, -6.9031) (21.5618, -6.8992) (21.5976, -6.8952) (21.6335, -6.891) (21.6694, -6.8867) (21.7053, -6.8822) (21.7412, -6.8776) (21.7771, -6.8729) (21.8131, -6.868) (21.8491, -6.863) (21.8851, -6.8578) (21.9139, -6.8536) (21.9356, -6.8503) (21.95, -6.8481) (21.9572, -6.847) knots 0.06937658 0.06937658 0.06937658 0.06937658 0.06937658 0.06937658 0.07142857 0.08571429 0.1 0.11428571 0.12857143 0.14285714 0.15714286 0.17142857 0.18571429 0.2 0.21428571 0.22857143 0.24285714 0.25714286 0.27142857 0.28571429 0.3 0.31428571 0.32857143 0.34285714 0.35714286 0.37142857 0.38571429 0.4 0.41428571 0.42857143 0.44285714 0.45714286 0.47142857 0.48571429 0.5 0.51428571 0.52857143 0.54285714 0.55714286 0.57142857 0.58571429 0.6 0.61428571 0.62857143 0.64285714 0.65714286 0.67142857 0.68571429 0.7 0.71428571 0.72857143 0.74285714 0.75714286 0.77142857 0.78571429 0.8 0.81428571 0.82857143 0.84285714 0.85714286 0.87142857 0.88571429 0.9 0.91428571 0.92857143 0.94285714 0.95714286 0.97142857 0.98571429 1 1 1 1 1 1
  arc A81 (21.9572, -6.847) -> (22.1733, -6.1109) centre (0, 0) ccw
  spline S102 degree 5 poles (22.1733, -6.1109) (22.1679, -6.106) (22.1569, -6.0964) (22.1405, -6.082) (22.1185, -6.0628) (22.091, -6.039) (22.0635, -6.0153) (22.0359, -5.9918) (22.0082, -5.9684) (21.9804, -5.9451) (21.9526, -5.9219) (21.9248, -5.8989) (21.8969, -5.876) (21.8689, -5.8532) (21.8409, -5.8306) (21.8128, -5.8081) (21.7846, -5.7857) (21.7564, -5.7635) (21.7281, -5.7414) (21.6998, -5.7194) (21.6714, -5.6976) (21.643, -5.6759) (21.6145, -5.6544) (21.5859, -5.633) (21.5573, -5.6118) (21.5286, -5.5907) (21.4999, -5.5697) (21.4711, -5.5489) (21.4422, -5.5283) (21.4133, -5.5078) (21.3843, -5.4874) (21.3552, -5.4672) (21.3261, -5.4472) (21.297, -5.4273) (21.2677, -5.4076) (21.2385, -5.3881) (21.2091, -5.3687) (21.1797, -5.3494) (21.1502, -5.3304) (21.1207, -5.3115) (21.0911, -5.2928) (21.0614, -5.2743) (21.0317, -5.2559) (21.0019, -5.2377) (20.972, -5.2197) (20.9421, -5.2019) (20.9121, -5.1843) (20.8821, -5.1668) (20.852, -5.1496) (20.8218, -5.1326) (20.7915, -5.1157) (20.7612, -5.0991) (20.7308, -5.0827) (20.7003, -5.0665) (20.6698, -5.0505) (20.6392, -5.0347) (20.6085, -5.0192) (20.5777, -5.004) (20.5469, -4.989) (20.516, -4.9742) (20.485, -4.9597) (20.4539, -4.9455) (20.4227, -4.9315) (20.3915, -4.9178) (20.3602, -4.9044) (20.3287, -4.8914) (20.3026, -4.8809) (20.2827, -4.8732) (20.2691, -4.8681) (20.2618, -4.8654) (20.2609, -4.865) knots -1 -1 -1 -1 -1 -1 -0.98571429 -0.97142857 -0.95714286 -0.94285714 -0.92857143 -0.91428571 -0.9 -0.88571429 -0.87142857 -0.85714286 -0.84285714 -0.82857143 -0.81428571 -0.8 -0.78571429 -0.77142857 -0.75714286 -0.74285714 -0.72857143 -0.71428571 -0.7 -0.68571429 -0.67142857 -0.65714286 -0.64285714 -0.62857143 -0.61428571 -0.6 -0.58571429 -0.57142857 -0.55714286 -0.54285714 -0.52857143 -0.51428571 -0.5 -0.48571429 -0.47142857 -0.45714286 -0.44285714 -0.42857143 -0.41428571 -0.4 -0.38571429 -0.37142857 -0.35714286 -0.34285714 -0.32857143 -0.31428571 -0.3 -0.28571429 -0.27142857 -0.25714286 -0.24285714 -0.22857143 -0.21428571 -0.2 -0.18571429 -0.17142857 -0.15714286 -0.14285714 -0.12857143 -0.11428571 -0.1 -0.08571429 -0.07142857 -0.06937658 -0.06937658 -0.06937658 -0.06937658 -0.06937658 -0.06937658
  spline S103 degree 3 poles (20.1986, -4.7484) (20.1956, -4.7611) (20.1951, -4.7743) (20.1992, -4.8) (20.2038, -4.8123) (20.2163, -4.8329) (20.2237, -4.8414) (20.2408, -4.8555) (20.2505, -4.8611) (20.2609, -4.865) knots 0 0 0 0 0.003906 0.003906 0.007813 0.007813 0.011148 0.011148 0.014483 0.014483 0.014483 0.014483
  arc A82 (20.1986, -4.7484) -> (20.3458, -4.0714) centre (0, 0) ccw
  spline S104 degree 3 poles (20.451, -3.9913) (20.438, -3.9904) (20.4249, -3.992) (20.4002, -4.0002) (20.3888, -4.0066) (20.3704, -4.0223) (20.3632, -4.0309) (20.352, -4.0501) (20.348, -4.0605) (20.3458, -4.0714) knots 0 0 0 0 0.003906 0.003906 0.007813 0.007813 0.011148 0.011148 0.014483 0.014483 0.014483 0.014483
  spline S105 degree 5 poles (20.451, -3.9913) (20.452, -3.9914) (20.4597, -3.9919) (20.4742, -3.9929) (20.4955, -3.9941) (20.5236, -3.9955) (20.5576, -3.9967) (20.5917, -3.9975) (20.6258, -3.9981) (20.6599, -3.9983) (20.6941, -3.9983) (20.7284, -3.9979) (20.7626, -3.9974) (20.7969, -3.9965) (20.8312, -3.9954) (20.8656, -3.9941) (20.9, -3.9924) (20.9344, -3.9906) (20.9688, -3.9885) (21.0033, -3.9862) (21.0378, -3.9837) (21.0723, -3.9809) (21.1068, -3.978) (21.1414, -3.9748) (21.176, -3.9714) (21.2106, -3.9679) (21.2452, -3.9641) (21.2798, -3.9601) (21.3145, -3.956) (21.3491, -3.9516) (21.3838, -3.9471) (21.4185, -3.9423) (21.4532, -3.9374) (21.488, -3.9323) (21.5227, -3.9271) (21.5575, -3.9216) (21.5922, -3.916) (21.627, -3.9102) (21.6618, -3.9042) (21.6966, -3.8981) (21.7314, -3.8918) (21.7662, -3.8854) (21.801, -3.8787) (21.8359, -3.8719) (21.8707, -3.865) (21.9056, -3.8579) (21.9404, -3.8506) (21.9753, -3.8432) (22.0101, -3.8356) (22.045, -3.8278) (22.0799, -3.8199) (22.1148, -3.8119) (22.1497, -3.8037) (22.1846, -3.7953) (22.2195, -3.7868) (22.2544, -3.7782) (22.2893, -3.7694) (22.3242, -3.7604) (22.3591, -3.7513) (22.394, -3.7421) (22.4289, -3.7327) (22.4638, -3.7232) (22.4987, -3.7135) (22.5336, -3.7037) (22.5685, -3.6937) (22.6034, -3.6837) (22.6383, -3.6734) (22.6662, -3.6651) (22.6872, -3.6588) (22.7011, -3.6546) (22.7081, -3.6525) knots 0.06937658 0.06937658 0.06937658 0.06937658 0.06937658 0.06937658 0.07142857 0.08571429 0.1 0.11428571 0.12857143 0.14285714 0.15714286 0.17142857 0.18571429 0.2 0.21428571 0.22857143 0.24285714 0.25714286 0.27142857 0.28571429 0.3 0.31428571 0.32857143 0.34285714 0.35714286 0.37142857 0.38571429 0.4 0.41428571 0.42857143 0.44285714 0.45714286 0.47142857 0.48571429 0.5 0.51428571 0.52857143 0.54285714 0.55714286 0.57142857 0.58571429 0.6 0.61428571 0.62857143 0.64285714 0.65714286 0.67142857 0.68571429 0.7 0.71428571 0.72857143 0.74285714 0.75714286 0.77142857 0.78571429 0.8 0.81428571 0.82857143 0.84285714 0.85714286 0.87142857 0.88571429 0.9 0.91428571 0.92857143 0.94285714 0.95714286 0.97142857 0.98571429 1 1 1 1 1 1
  arc A83 (22.7081, -3.6525) -> (22.8173, -2.8931) centre (0, 0) ccw
  spline S106 degree 5 poles (22.8173, -2.8931) (22.8112, -2.8891) (22.799, -2.8811) (22.7807, -2.8692) (22.7562, -2.8533) (22.7256, -2.8337) (22.695, -2.8142) (22.6643, -2.7948) (22.6336, -2.7755) (22.6028, -2.7564) (22.572, -2.7374) (22.5411, -2.7186) (22.5102, -2.6999) (22.4793, -2.6814) (22.4483, -2.6629) (22.4173, -2.6447) (22.3863, -2.6265) (22.3552, -2.6085) (22.3241, -2.5907) (22.2929, -2.573) (22.2617, -2.5554) (22.2305, -2.538) (22.1992, -2.5208) (22.1679, -2.5037) (22.1365, -2.4867) (22.1051, -2.4699) (22.0737, -2.4533) (22.0422, -2.4368) (22.0107, -2.4205) (21.9792, -2.4043) (21.9476, -2.3883) (21.9159, -2.3724) (21.8843, -2.3567) (21.8526, -2.3412) (21.8209, -2.3259) (21.7891, -2.3107) (21.7573, -2.2957) (21.7254, -2.2808) (21.6935, -2.2661) (21.6616, -2.2517) (21.6296, -2.2373) (21.5976, -2.2232) (21.5656, -2.2093) (21.5335, -2.1955) (21.5014, -2.1819) (21.4693, -2.1686) (21.4371, -2.1554) (21.4048, -2.1424) (21.3726, -2.1296) (21.3403, -2.1171) (21.3079, -2.1047) (21.2755, -2.0926) (21.2431, -2.0807) (21.2107, -2.069) (21.1782, -2.0575) (21.1456, -2.0462) (21.113, -2.0352) (21.0804, -2.0245) (21.0478, -2.0141) (21.0151, -2.0039) (20.9823, -1.9939) (20.9495, -1.9842) (20.9167, -1.9748) (20.8838, -1.9657) (20.8509, -1.9569) (20.8179, -1.9485) (20.7906, -1.9419) (20.7698, -1.9371) (20.7556, -1.9339) (20.748, -1.9323) (20.7471, -1.9321) knots -1 -1 -1 -1 -1 -1 -0.98571429 -0.97142857 -0.95714286 -0.94285714 -0.92857143 -0.91428571 -0.9 -0.88571429 -0.87142857 -0.85714286 -0.84285714 -0.82857143 -0.81428571 -0.8 -0.78571429 -0.77142857 -0.75714286 -0.74285714 -0.72857143 -0.71428571 -0.7 -0.68571429 -0.67142857 -0.65714286 -0.64285714 -0.62857143 -0.61428571 -0.6 -0.58571429 -0.57142857 -0.55714286 -0.54285714 -0.52857143 -0.51428571 -0.5 -0.48571429 -0.47142857 -0.45714286 -0.44285714 -0.42857143 -0.41428571 -0.4 -0.38571429 -0.37142857 -0.35714286 -0.34285714 -0.32857143 -0.31428571 -0.3 -0.28571429 -0.27142857 -0.25714286 -0.24285714 -0.22857143 -0.21428571 -0.2 -0.18571429 -0.17142857 -0.15714286 -0.14285714 -0.12857143 -0.11428571 -0.1 -0.08571429 -0.07142857 -0.06937658 -0.06937658 -0.06937658 -0.06937658 -0.06937658 -0.06937658
  spline S107 degree 3 poles (20.6687, -1.8256) (20.6676, -1.8385) (20.669, -1.8516) (20.6767, -1.8765) (20.683, -1.888) (20.6984, -1.9066) (20.7068, -1.914) (20.7258, -1.9255) (20.7362, -1.9297) (20.7471, -1.9321) knots 0 0 0 0 0.003906 0.003906 0.007813 0.007813 0.011148 0.011148 0.014483 0.014483 0.014483 0.014483
  arc A84 (20.6687, -1.8256) -> (20.7182, -1.1345) centre (0, 0) ccw
  spline S108 degree 3 poles (20.8108, -1.0402) (20.7979, -1.0411) (20.7852, -1.0446) (20.7619, -1.0562) (20.7514, -1.0642) (20.7355, -1.0824) (20.7296, -1.0919) (20.7212, -1.1125) (20.7188, -1.1234) (20.7182, -1.1345) knots 0 0 0 0 0.003906 0.003906 0.007813 0.007813 0.011148 0.011148 0.014483 0.014483 0.014483 0.014483
  spline S109 degree 5 poles (20.8108, -1.0402) (20.8118, -1.0401) (20.8195, -1.0396) (20.834, -1.0385) (20.8553, -1.0367) (20.8833, -1.034) (20.9172, -1.0304) (20.951, -1.0264) (20.9848, -1.022) (21.0187, -1.0174) (21.0525, -1.0125) (21.0863, -1.0073) (21.1202, -1.0019) (21.154, -0.9961) (21.1878, -0.9902) (21.2216, -0.9839) (21.2554, -0.9774) (21.2892, -0.9707) (21.323, -0.9637) (21.3568, -0.9565) (21.3906, -0.9491) (21.4244, -0.9415) (21.4581, -0.9337) (21.4919, -0.9256) (21.5256, -0.9174) (21.5594, -0.9089) (21.5931, -0.9002) (21.6268, -0.8914) (21.6605, -0.8823) (21.6942, -0.8731) (21.7279, -0.8636) (21.7616, -0.854) (21.7952, -0.8442) (21.8289, -0.8343) (21.8625, -0.8241) (21.8961, -0.8138) (21.9298, -0.8033) (21.9634, -0.7926) (21.9969, -0.7817) (22.0305, -0.7707) (22.0641, -0.7595) (22.0976, -0.7481) (22.1311, -0.7366) (22.1646, -0.7249) (22.1981, -0.7131) (22.2316, -0.7011) (22.2651, -0.6889) (22.2985, -0.6766) (22.332, -0.6642) (22.3654, -0.6515) (22.3988, -0.6387) (22.4322, -0.6258) (22.4655, -0.6127) (22.4989, -0.5995) (22.5322, -0.5861) (22.5655, -0.5726) (22.5988, -0.5589) (22.6321, -0.5451) (22.6653, -0.5311) (22.6986, -0.517) (22.7318, -0.5027) (22.765, -0.4883) (22.7982, -0.4738) (22.8313, -0.4591) (22.8645, -0.4443) (22.8976, -0.4294) (22.9307, -0.4143) (22.9571, -0.4021) (22.977, -0.3929) (22.9902, -0.3867) (22.9968, -0.3836) knots 0.06937658 0.06937658 0.06937658 0.06937658 0.06937658 0.06937658 0.07142857 0.08571429 0.1 0.11428571 0.12857143 0.14285714 0.15714286 0.17142857 0.18571429 0.2 0.21428571 0.22857143 0.24285714 0.25714286 0.27142857 0.28571429 0.3 0.31428571 0.32857143 0.34285714 0.35714286 0.37142857 0.38571429 0.4 0.41428571 0.42857143 0.44285714 0.45714286 0.47142857 0.48571429 0.5 0.51428571 0.52857143 0.54285714 0.55714286 0.57142857 0.58571429 0.6 0.61428571 0.62857143 0.64285714 0.65714286 0.67142857 0.68571429 0.7 0.71428571 0.72857143 0.74285714 0.75714286 0.77142857 0.78571429 0.8 0.81428571 0.82857143 0.84285714 0.85714286 0.87142857 0.88571429 0.9 0.91428571 0.92857143 0.94285714 0.95714286 0.97142857 0.98571429 1 1 1 1 1 1
  arc A85 (22.9968, -0.3836) -> (22.9968, 0.3836) centre (0, 0) ccw
  spline S110 degree 5 poles (22.9968, 0.3836) (22.9902, 0.3867) (22.977, 0.3929) (22.9571, 0.4021) (22.9307, 0.4143) (22.8976, 0.4294) (22.8645, 0.4443) (22.8313, 0.4591) (22.7982, 0.4738) (22.765, 0.4883) (22.7318, 0.5027) (22.6986, 0.517) (22.6653, 0.5311) (22.6321, 0.5451) (22.5988, 0.5589) (22.5655, 0.5726) (22.5322, 0.5861) (22.4989, 0.5995) (22.4655, 0.6127) (22.4322, 0.6258) (22.3988, 0.6387) (22.3654, 0.6515) (22.332, 0.6642) (22.2985, 0.6766) (22.2651, 0.6889) (22.2316, 0.7011) (22.1981, 0.7131) (22.1646, 0.7249) (22.1311, 0.7366) (22.0976, 0.7481) (22.0641, 0.7595) (22.0305, 0.7707) (21.9969, 0.7817) (21.9634, 0.7926) (21.9298, 0.8033) (21.8961, 0.8138) (21.8625, 0.8241) (21.8289, 0.8343) (21.7952, 0.8442) (21.7616, 0.854) (21.7279, 0.8636) (21.6942, 0.8731) (21.6605, 0.8823) (21.6268, 0.8914) (21.5931, 0.9002) (21.5594, 0.9089) (21.5256, 0.9174) (21.4919, 0.9256) (21.4581, 0.9337) (21.4244, 0.9415) (21.3906, 0.9491) (21.3568, 0.9565) (21.323, 0.9637) (21.2892, 0.9707) (21.2554, 0.9774) (21.2216, 0.9839) (21.1878, 0.9902) (21.154, 0.9961) (21.1202, 1.0019) (21.0863, 1.0073) (21.0525, 1.0125) (21.0187, 1.0174) (20.9848, 1.022) (20.951, 1.0264) (20.9172, 1.0304) (20.8833, 1.034) (20.8553, 1.0367) (20.834, 1.0385) (20.8195, 1.0396) (20.8118, 1.0401) (20.8108, 1.0402) knots -1 -1 -1 -1 -1 -1 -0.98571429 -0.97142857 -0.95714286 -0.94285714 -0.92857143 -0.91428571 -0.9 -0.88571429 -0.87142857 -0.85714286 -0.84285714 -0.82857143 -0.81428571 -0.8 -0.78571429 -0.77142857 -0.75714286 -0.74285714 -0.72857143 -0.71428571 -0.7 -0.68571429 -0.67142857 -0.65714286 -0.64285714 -0.62857143 -0.61428571 -0.6 -0.58571429 -0.57142857 -0.55714286 -0.54285714 -0.52857143 -0.51428571 -0.5 -0.48571429 -0.47142857 -0.45714286 -0.44285714 -0.42857143 -0.41428571 -0.4 -0.38571429 -0.37142857 -0.35714286 -0.34285714 -0.32857143 -0.31428571 -0.3 -0.28571429 -0.27142857 -0.25714286 -0.24285714 -0.22857143 -0.21428571 -0.2 -0.18571429 -0.17142857 -0.15714286 -0.14285714 -0.12857143 -0.11428571 -0.1 -0.08571429 -0.07142857 -0.06937658 -0.06937658 -0.06937658 -0.06937658 -0.06937658 -0.06937658
  spline S111 degree 3 poles (20.7182, 1.1345) (20.7189, 1.1215) (20.7221, 1.1087) (20.7333, 1.0852) (20.7411, 1.0747) (20.759, 1.0584) (20.7684, 1.0524) (20.7889, 1.0436) (20.7998, 1.041) (20.8108, 1.0402) knots 0 0 0 0 0.003906 0.003906 0.007813 0.007813 0.011148 0.011148 0.014483 0.014483 0.014483 0.014483
  arc A86 (20.7182, 1.1345) -> (20.6687, 1.8256) centre (0, 0) ccw
  spline S112 degree 3 poles (20.7471, 1.9321) (20.7343, 1.9293) (20.7223, 1.9241) (20.7008, 1.9093) (20.6917, 1.8999) (20.6785, 1.8796) (20.674, 1.8694) (20.6686, 1.8478) (20.6678, 1.8366) (20.6687, 1.8256) knots 0 0 0 0 0.003906 0.003906 0.007813 0.007813 0.011148 0.011148 0.014483 0.014483 0.014483 0.014483
  spline S113 degree 5 poles (20.7471, 1.9321) (20.748, 1.9323) (20.7556, 1.9339) (20.7698, 1.9371) (20.7906, 1.9419) (20.8179, 1.9485) (20.8509, 1.9569) (20.8838, 1.9657) (20.9167, 1.9748) (20.9495, 1.9842) (20.9823, 1.9939) (21.0151, 2.0039) (21.0478, 2.0141) (21.0804, 2.0245) (21.113, 2.0352) (21.1456, 2.0462) (21.1782, 2.0575) (21.2107, 2.069) (21.2431, 2.0807) (21.2755, 2.0926) (21.3079, 2.1047) (21.3403, 2.1171) (21.3726, 2.1296) (21.4048, 2.1424) (21.4371, 2.1554) (21.4693, 2.1686) (21.5014, 2.1819) (21.5335, 2.1955) (21.5656, 2.2093) (21.5976, 2.2232) (21.6296, 2.2373) (21.6616, 2.2517) (21.6935, 2.2661) (21.7254, 2.2808) (21.7573, 2.2957) (21.7891, 2.3107) (21.8209, 2.3259) (21.8526, 2.3412) (21.8843, 2.3567) (21.9159, 2.3724) (21.9476, 2.3883) (21.9792, 2.4043) (22.0107, 2.4205) (22.0422, 2.4368) (22.0737, 2.4533) (22.1051, 2.4699) (22.1365, 2.4867) (22.1679, 2.5037) (22.1992, 2.5208) (22.2305, 2.538) (22.2617, 2.5554) (22.2929, 2.573) (22.3241, 2.5907) (22.3552, 2.6085) (22.3863, 2.6265) (22.4173, 2.6447) (22.4483, 2.6629) (22.4793, 2.6814) (22.5102, 2.6999) (22.5411, 2.7186) (22.572, 2.7374) (22.6028, 2.7564) (22.6336, 2.7755) (22.6643, 2.7948) (22.695, 2.8142) (22.7256, 2.8337) (22.7562, 2.8533) (22.7807, 2.8692) (22.799, 2.8811) (22.8112, 2.8891) (22.8173, 2.8931) knots 0.06937658 0.06937658 0.06937658 0.06937658 0.06937658 0.06937658 0.07142857 0.08571429 0.1 0.11428571 0.12857143 0.14285714 0.15714286 0.17142857 0.18571429 0.2 0.21428571 0.22857143 0.24285714 0.25714286 0.27142857 0.28571429 0.3 0.31428571 0.32857143 0.34285714 0.35714286 0.37142857 0.38571429 0.4 0.41428571 0.42857143 0.44285714 0.45714286 0.47142857 0.48571429 0.5 0.51428571 0.52857143 0.54285714 0.55714286 0.57142857 0.58571429 0.6 0.61428571 0.62857143 0.64285714 0.65714286 0.67142857 0.68571429 0.7 0.71428571 0.72857143 0.74285714 0.75714286 0.77142857 0.78571429 0.8 0.81428571 0.82857143 0.84285714 0.85714286 0.87142857 0.88571429 0.9 0.91428571 0.92857143 0.94285714 0.95714286 0.97142857 0.98571429 1 1 1 1 1 1
  arc A87 (22.8173, 2.8931) -> (22.7081, 3.6525) centre (0, 0) ccw
  spline S114 degree 5 poles (22.7081, 3.6525) (22.7011, 3.6546) (22.6872, 3.6588) (22.6662, 3.6651) (22.6383, 3.6734) (22.6034, 3.6837) (22.5685, 3.6937) (22.5336, 3.7037) (22.4987, 3.7135) (22.4638, 3.7232) (22.4289, 3.7327) (22.394, 3.7421) (22.3591, 3.7513) (22.3242, 3.7604) (22.2893, 3.7694) (22.2544, 3.7782) (22.2195, 3.7868) (22.1846, 3.7953) (22.1497, 3.8037) (22.1148, 3.8119) (22.0799, 3.8199) (22.045, 3.8278) (22.0101, 3.8356) (21.9753, 3.8432) (21.9404, 3.8506) (21.9056, 3.8579) (21.8707, 3.865) (21.8359, 3.8719) (21.801, 3.8787) (21.7662, 3.8854) (21.7314, 3.8918) (21.6966, 3.8981) (21.6618, 3.9042) (21.627, 3.9102) (21.5922, 3.916) (21.5575, 3.9216) (21.5227, 3.9271) (21.488, 3.9323) (21.4532, 3.9374) (21.4185, 3.9423) (21.3838, 3.9471) (21.3491, 3.9516) (21.3145, 3.956) (21.2798, 3.9601) (21.2452, 3.9641) (21.2106, 3.9679) (21.176, 3.9714) (21.1414, 3.9748) (21.1068, 3.978) (21.0723, 3.9809) (21.0378, 3.9837) (21.0033, 3.9862) (20.9688, 3.9885) (20.9344, 3.9906) (20.9, 3.9924) (20.8656, 3.9941) (20.8312, 3.9954) (20.7969, 3.9965) (20.7626, 3.9974) (20.7284, 3.9979) (20.6941, 3.9983) (20.6599, 3.9983) (20.6258, 3.9981) (20.5917, 3.9975) (20.5576, 3.9967) (20.5236, 3.9955) (20.4955, 3.9941) (20.4742, 3.9929) (20.4597, 3.9919) (20.452, 3.9914) (20.451, 3.9913) knots -1 -1 -1 -1 -1 -1 -0.98571429 -0.97142857 -0.95714286 -0.94285714 -0.92857143 -0.91428571 -0.9 -0.88571429 -0.87142857 -0.85714286 -0.84285714 -0.82857143 -0.81428571 -0.8 -0.78571429 -0.77142857 -0.75714286 -0.74285714 -0.72857143 -0.71428571 -0.7 -0.68571429 -0.67142857 -0.65714286 -0.64285714 -0.62857143 -0.61428571 -0.6 -0.58571429 -0.57142857 -0.55714286 -0.54285714 -0.52857143 -0.51428571 -0.5 -0.48571429 -0.47142857 -0.45714286 -0.44285714 -0.42857143 -0.41428571 -0.4 -0.38571429 -0.37142857 -0.35714286 -0.34285714 -0.32857143 -0.31428571 -0.3 -0.28571429 -0.27142857 -0.25714286 -0.24285714 -0.22857143 -0.21428571 -0.2 -0.18571429 -0.17142857 -0.15714286 -0.14285714 -0.12857143 -0.11428571 -0.1 -0.08571429 -0.07142857 -0.06937658 -0.06937658 -0.06937658 -0.06937658 -0.06937658 -0.06937658
  spline S115 degree 3 poles (20.3458, 4.0714) (20.3484, 4.0587) (20.3534, 4.0465) (20.3678, 4.0248) (20.3771, 4.0155) (20.3971, 4.002) (20.4073, 3.9973) (20.4287, 3.9916) (20.4399, 3.9905) (20.451, 3.9913) knots 0 0 0 0 0.003906 0.003906 0.007813 0.007813 0.011148 0.011148 0.014483 0.014483 0.014483 0.014483
  arc A88 (20.3458, 4.0714) -> (20.1986, 4.7484) centre (0, 0) ccw
  spline S116 degree 3 poles (20.2609, 4.865) (20.2487, 4.8605) (20.2375, 4.8536) (20.2184, 4.8359) (20.2107, 4.8252) (20.2005, 4.8034) (20.1975, 4.7926) (20.1953, 4.7704) (20.196, 4.7593) (20.1986, 4.7484) knots 0 0 0 0 0.003906 0.003906 0.007813 0.007813 0.011148 0.011148 0.014483 0.014483 0.014483 0.014483